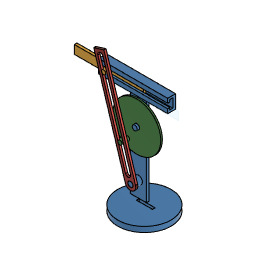
Crank and slotted link mechanism v5 (Autodesk Fusion 360 design; units mm, degrees)
Autodesk Fusion 360 part; units mm, degrees
note: some values were not read from the file. Chosen so that the rebuilt part matches the saved one: which face or edge a step refers to.
sketch "Holder stand" plane through (0, 0, 0) normal (0, 0, 1) x (1, 0, 0)
  circle A0 centre (0, 0) radius 50
  dimension "d1" = 100
  constraint coincident A0.centre origin
  measures "d1" diameter of A0
extrude "Extrude1" add sketch "Holder stand" along normal blind 10 makes body 1
sketch "Holder" plane through (0, 0, 10) normal (0, 0, 1) x (-1, 0, 0)
  circle A0 centre (0, 0) radius 50
  line L0 (0, 0) -> (-15, 0)
  line L1 (-15, 0) -> (-15, -5)
  line L2 (-15, -5) -> (0, -5)
  line L3 (0, -5) -> (0, 0)
  line L4 (15, -5) -> (0, -5)
  line L5 (15, 0) -> (15, -5)
  line L6 (0, 0) -> (15, 0)
  dimension "d4" = 15
  dimension "d5" = 5
  constraint horizontal L0
  constraint vertical L1
  constraint horizontal L2
  constraint vertical L3
  constraint coincident A0.centre L0.start
  constraint symmetric A0.centre L3 L0.start
  constraint symmetric L0.end L3 L5.start
  constraint symmetric L1.end L3 L4.start
  constraint symmetric L2.end L3 L4.end
  measures "d4" distance of A0.centre L0.end
  measures "d5" distance of A0.centre L2.end
extrude "Extrude2" cut sketch "Holder" against normal blind 10 contours L0 L1 L2 L3 | L3 L4 L5 L6 bodies 1
extrude "Extrude3" add sketch "Holder" along normal blind 190 separate body contours L0 L1 L2 L3 | L3 L4 L5 L6 makes body 2
extrude "Extrude4" add 1 faces at (10, 1.6667, 10) along direction (0, 0, -1) blind 10 on bodies 2 bodies 2
sketch "Crank Holder" plane through (0, 0, 0) normal (0, -1, 0) x (1, 0, 0)
  line L0 (15, 0) -> (15, 200)
  line L1 (15, 200) -> (-15, 200)
  line L2 (-15, 200) -> (-15, 0)
  line L3 (-15, 0) -> (15, 0)
  line L4 (0, 200) -> (0, 118)
  circle A0 centre (0, 118) radius 5
  dimension "d12" = 82
  dimension "d13" = 10
  constraint midpoint L1 L4.start
  constraint perpendicular L1 L4
  constraint coincident L4.end A0.centre
  measures "d12" distance of L4.start L4.end
  measures "d13" diameter of A0
extrude "Extrude5" add sketch "Crank Holder" along normal blind 7 contours A0 bodies 2
sketch "Crank" plane through (0, 0, 0) normal (0, -1, 0) x (1, 0, 0)
  circle A0 centre (0, 118) radius 5
  line L0 (15, 0) -> (15, 200)
  line L1 (15, 200) -> (-15, 200)
  line L2 (-15, 200) -> (-15, 0)
  line L3 (-15, 0) -> (15, 0)
  circle A1 centre (0, 118) radius 45
  dimension "d16" = 90
  constraint concentric A0 A1
  measures "d16" diameter of A1
extrude "Extrude6" add sketch "Crank" along normal blind 3 separate body contours A0 | L0 L2 A1 | L0 A1 | L2 A1 makes body 3
extrude "Extrude7" cut sketch "Crank Holder" along normal blind 9 contours A0 bodies 3
move_face "OffsetFaces1" offset -0.3 1 faces at (4.9938, -2.3333, 118.2492) on bodies 2
sketch "slider holder right" plane through (15, 0, 0) normal (1, 0, 0) x (0, 1, 0)
  line L0 (5, 0) -> (5, 200)
  line L1 (5, 200) -> (0, 200)
  line L2 (0, 200) -> (0, 0)
  line L3 (0, 0) -> (5, 0)
  line L4 (0, 200) -> (5, 200)
  line L5 (5, 200) -> (5, 175)
  line L6 (5, 175) -> (0, 175)
  line L7 (0, 175) -> (0, 200)
  dimension "d22" = 5
  dimension "d23" = 25
  constraint horizontal L4
  constraint vertical L5
  constraint horizontal L6
  constraint vertical L7
  constraint coincident L1.end L2.start
  measures "d22" distance of L1.end L0.end
  measures "d23" distance of L1.end L6.end
sketch "slider holder left" plane through (-15, 0, 0) normal (-1, 0, 0) x (0, -1, 0)
  line L0 (0, 0) -> (0, 200)
  line L1 (0, 200) -> (-5, 200)
  line L2 (-5, 200) -> (-5, 0)
  line L3 (-5, 0) -> (0, 0)
  line L4 (-5, 200) -> (0, 200)
  line L5 (0, 200) -> (0, 175)
  line L6 (0, 175) -> (-5, 175)
  line L7 (-5, 175) -> (-5, 200)
  constraint horizontal L4
  constraint vertical L5
  constraint horizontal L6
  constraint vertical L7
  constraint coincident L0 L5.end
  constraint coincident L1.end L2.start
extrude "Extrude8" add sketch "slider holder left" along normal blind 50 contours L0 L1 L2 L4 L5 L6 L7 bodies 2
extrude "Extrude9" add sketch "slider holder right" along normal blind 50 contours L0 L1 L2 L4 L5 L6 L7 bodies 2
sketch "slider holder front" plane through (0, 0, 0) normal (0, -1, 0) x (1, 0, 0)
  circle A0 centre (0, 118) radius 4.7
  line L0 (65, 200) -> (-65, 200)
  line L1 (-65, 200) -> (-65, 175)
  line L2 (-65, 175) -> (-15, 175)
  line L3 (-15, 175) -> (-15, 0)
  line L4 (-15, 0) -> (15, 0)
  line L5 (15, 0) -> (15, 175)
  line L6 (15, 175) -> (65, 175)
  line L7 (65, 175) -> (65, 200)
  line L8 (-65, 200) -> (65, 200)
  line L9 (65, 200) -> (65, 196)
  line L10 (65, 196) -> (-65, 196)
  line L11 (-65, 196) -> (-65, 200)
  line L12 (-65, 175) -> (65, 175)
  line L13 (65, 175) -> (65, 179)
  line L14 (65, 179) -> (-65, 179)
  line L15 (-65, 179) -> (-65, 175)
  dimension "d28" = 4
  dimension "d29" = 4
  constraint horizontal L8
  constraint vertical L9
  constraint horizontal L10
  constraint vertical L11
  constraint coincident L7 L9.end
  constraint coincident L0.end L1.start
  constraint horizontal L12
  constraint vertical L13
  constraint horizontal L14
  constraint vertical L15
  constraint coincident L7 L13.end
  constraint coincident L1.end L2.start
  measures "d28" distance of L0.end L10.end
  measures "d29" distance of L1.end L14.end
extrude "Extrude10" add sketch "slider holder front" along normal blind 10 contours L0 L1 L7 L8 L9 L10 L11 | L1 L2 L6 L7 L12 L13 L14 L15 bodies 2
sketch "slider barrier top" plane through (0, 0, 179) normal (0, 0, 1) x (-1, 0, 0)
  line L0 (-65, 0) -> (65, 0)
  line L1 (65, 0) -> (65, 10)
  line L2 (65, 10) -> (-65, 10)
  line L3 (-65, 10) -> (-65, 0)
  line L4 (65, 10) -> (-65, 10)
  line L5 (-65, 10) -> (-65, 6)
  line L6 (-65, 6) -> (65, 6)
  line L7 (65, 6) -> (65, 10)
  dimension "d32" = 4
  constraint horizontal L4
  constraint vertical L5
  constraint horizontal L6
  constraint vertical L7
  constraint coincident L3 L5.end
  constraint coincident L1.end L2.start
  measures "d32" distance of L1.end L6.end
sketch "slider barrier bottom" plane through (0, 0, 196) normal (0, 0, -1) x (1, 0, 0)
  line L0 (-65, 0) -> (65, 0)
  line L1 (65, 0) -> (65, 10)
  line L2 (65, 10) -> (-65, 10)
  line L3 (-65, 10) -> (-65, 0)
  line L4 (-65, 10) -> (65, 10)
  line L5 (65, 10) -> (65, 6)
  line L6 (65, 6) -> (-65, 6)
  line L7 (-65, 6) -> (-65, 10)
  dimension "d33" = 4
  constraint horizontal L4
  constraint vertical L5
  constraint horizontal L6
  constraint vertical L7
  constraint coincident L1 L5.end
  constraint coincident L2.end L3.start
  measures "d33" distance of L2.end L6.end
extrude "Extrude11" add sketch "slider barrier bottom" along normal blind 4 contours L1 L2 L3 L4 L5 L6 L7 bodies 2
extrude "Extrude12" add sketch "slider barrier top" along normal blind 4 contours L1 L2 L3 L4 L5 L6 L7 bodies 2
sketch "slider" plane through (65, 0, 0) normal (1, 0, 0) x (0, 1, 0)
  line L0 (-10, 175) -> (5, 175)
  line L1 (5, 175) -> (5, 200)
  line L2 (5, 200) -> (-10, 200)
  line L3 (-10, 200) -> (-10, 192)
  line L4 (-10, 192) -> (-6, 192)
  line L5 (-6, 192) -> (-6, 196)
  line L6 (-6, 196) -> (0, 196)
  line L7 (0, 196) -> (0, 179)
  line L8 (0, 179) -> (-6, 179)
  line L9 (-6, 179) -> (-6, 183)
  line L10 (-6, 183) -> (-10, 183)
  line L11 (-10, 183) -> (-10, 175)
  line L12 (-6, 196) -> (0, 196)
  line L13 (0, 196) -> (0, 179)
  line L14 (0, 179) -> (-6, 179)
  line L15 (-6, 179) -> (-6, 196)
  constraint horizontal L12
  constraint vertical L13
  constraint horizontal L14
  constraint vertical L15
  constraint coincident L7.end L8.start
  constraint coincident L5.end L6.start
extrude "Extrude13" add sketch "slider" against normal blind 130 separate body contours L5 L6 L7 L8 L9 L12 L13 L14 L15 makes body 4
move_face "OffsetFaces4" offset -0.3 7 faces at (21.6667, -6, 186) (-21.6667, -6, 193.3333) (21.6667, -4, 196) (-21.6667, 0, 190.3333) (21.6667, -2, 179) (-21.6667, -6, 180.3333) (65, -2, 186) on bodies 4
move_face "OffsetFaces2" offset -0.3 5 faces at (21.4667, -5.7, 186) (21.4667, -5.7, 193.2333) (21.4667, -5.7, 180.5333) (21.4667, -3.9, 195.7) (21.4667, -0.3, 190.2333) on bodies 4
sketch "link holder" plane through (0, 0, 0) normal (0, -1, 0) x (1, 0, 0)
  circle A0 centre (0, 118) radius 4.7
  line L0 (15, 175) -> (-15, 175)
  line L1 (-15, 175) -> (-15, 0)
  line L2 (-15, 0) -> (15, 0)
  line L3 (15, 0) -> (15, 175)
  circle A1 centre (0, 30) radius 5
  dimension "d41" = 10
  measures "d41" diameter of A1
extrude "Extrude14" add sketch "link holder" along normal blind 15 contours A1 bodies 2
sketch "slotted link" plane through (0, -15, 0) normal (0, -1, 0) x (1, 0, 0)
  circle A0 centre (0, 30) radius 5
  circle A1 centre (0, 30) radius 10
  line L0 (-10, 30) -> (10, 30)
  line L1 (-10, 30) -> (10, 30)
  line L2 (10, 30) -> (10, 230)
  line L3 (10, 230) -> (-10, 230)
  line L4 (-10, 230) -> (-10, 30)
  line L5 (-5, 30) -> (5, 30)
  line L6 (5, 30) -> (5, 225)
  line L7 (5, 225) -> (-5, 225)
  line L8 (-5, 225) -> (-5, 30)
  circle A2 centre (0, 45) radius 5
  circle A3 centre (0, 220) radius 5
  dimension "d44" = 5
  dimension "d45" = 20
  dimension "d46" = 200
  dimension "d47" = 195
  dimension "d48" = 10
  constraint coincident A1 L0.start
  constraint coincident A1 L0.end
  constraint horizontal L0
  constraint horizontal L1
  constraint vertical L2
  constraint horizontal L3
  constraint vertical L4
  constraint horizontal L5
  constraint vertical L6
  constraint horizontal L7
  constraint vertical L8
  constraint coincident L0 L5.start
  constraint coincident A0 L5.start
  constraint tangent L7 A3
  constraint tangent L6 A3
  measures "d44" distance of A0
  measures "d45" distance of L0.start L0.end
  measures "d46" distance of L0.start L3.end
  measures "d47" distance of L5.start L7.end
  measures "d48" diameter of A2
extrude "Extrude15" add sketch "slotted link" against normal blind 4 separate body contours A0 A1 L0 L1 | A1 L0 L1 L6 | A0 A1 L6 L8 | A1 L0 L1 L8 | A1 L2 L3 L4 L6 L7 L8 | A1 L6 A2 | A1 L8 A2 | L6 L7 A3 | L7 L8 A3 makes body 5
move_face "OffsetFaces3" offset -0.3 1 faces at (4.9752, -10, 29.5022) on bodies 2
sketch "slotted link holder" plane through (0, -15, 0) normal (0, -1, 0) x (1, 0, 0)
  circle A0 centre (0, 30) radius 4.7
  circle A1 centre (0, 30) radius 7.5
  dimension "d52" = 15
  constraint concentric A0 A1
  measures "d52" diameter of A1
extrude "Extrude16" add sketch "slotted link holder" along normal blind -15 and the other way blind 4 bodies 2
sketch "crank pin" plane through (0, -3, 0) normal (0, -1, 0) x (1, 0, 0)
  circle A0 centre (0, 118) radius 5
  circle A1 centre (0, 118) radius 45
  circle A2 centre (0, 85) radius 4
  dimension "d57" = 8
  measures "d57" diameter of A2
sketch "slider modif" plane through (0, -0.6, 0) normal (0, 1, 0) x (-1, 0, 0)
  line L0 (-64.7, 195.4) -> (-64.7, 179.3)
  line L1 (-64.7, 179.3) -> (65, 179.3)
  line L2 (65, 179.3) -> (65, 195.4)
  line L3 (65, 195.4) -> (-64.7, 195.4)
sketch "slider pin (1)" plane through (0, -5.4, 0) normal (0, -1, 0) x (1, 0, 0)
  line L0 (64.7, 179.3) -> (64.7, 195.4)
  line L1 (64.7, 195.4) -> (-65, 195.4)
  line L2 (-65, 195.4) -> (-65, 179.3)
  line L3 (-65, 179.3) -> (64.7, 179.3)
  circle A0 centre (-0.0455, 187.5901) radius 4
  dimension "d64" = 8
  measures "d64" diameter of A0
extrude "Extrude18" add sketch "slider pin (1)" along normal blind 10 contours A0 bodies 4
extrude "Extrude19" add sketch "crank pin" along normal blind 14 contours A2 bodies 3
copy_body "Body->Comp1" bodies 1 removing the originals makes body 6 in component "Holder stand"
copy_body "Body->Comp2" bodies 3 removing the originals makes body 7 in component "Crank"
copy_body "Body->Comp3" bodies 4 removing the originals makes body 8 in component "Slider"
copy_body "Body->Comp4" bodies 5 removing the originals makes body 9 in component "Slotted Link"
copy_body "Body->Comp5" bodies 2 removing the originals makes body 10 in component "Holder"
extrude "Extrude17" [suppressed]
sketch "slider pin" plane through (0, -5.4, 0) normal (0, -1, 0) x (1, 0, 0)
  line L0 (64.7, 179.3) -> (64.7, 195.4)
  line L1 (64.7, 195.4) -> (-65, 195.4)
  line L2 (-65, 195.4) -> (-65, 179.3)
  circle A0 centre (0, 187.5) radius 4
  circle A1 centre (0, 187.5) radius 4
  line L3 (-65, 179.3) -> (64.7, 179.3)
  dimension "d58" = 8
  measures "d58" diameter of A0
component "Holder stand" placed x (1, 0, 0) y (0, 1, 0) z (0, 0, 1) at (0, 0, 0)
component "Crank" placed x (1, 0, 0) y (0, 1, 0) z (0, 0, 1) at (0, 0, 0)
component "Slider" placed x (1, 0, 0) y (0, 1, 0) z (0, 0, 1) at (0, 0, 0)
component "Slotted Link" placed x (1, 0, 0) y (0, 1, 0) z (0, 0, 1) at (0, 0, 0)
component "Holder" placed x (1, 0, 0) y (0, 1, 0) z (0, 0, 1) at (0, 0, 0)
named bodies: "Holder stand", "Holder", "Crank", "Slider", "Slotted Link"
